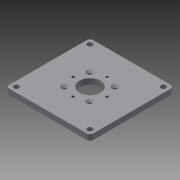
# Autodesk Inventor part: base_mount
Saved by Autodesk Inventor 2015 (Build 190159000, 159)
## iProperties
Created: 2015-12-01
Part Number: base_mount
Material: Generic
Document SubType Name: Modeling
Designer: jufranz
Density: 1 g/cm^3
Appearance: Default
Author: jufranz
Autodesk Inventor part; units mm, degrees
ref_plane "YZ Plane" through (0, 0, 0) normal (1, 0, 0) x (0, 1, 0)
ref_plane "XZ Plane" through (0, 0, 0) normal (0, 1, 0) x (-1, 0, 0)
ref_plane "XY Plane" through (0, 0, 0) normal (0, 0, 1) x (1, 0, 0)
sketch "Sketch1" plane through (0, 0, 0) normal (0, 1, 0) x (-1, 0, 0)
  line L0 (40, 36.825) -> (40, -36.825)
  line L1 (36.825, -40) -> (-36.825, -40)
  line L2 (-40, -36.825) -> (-40, 36.825)
  line L3 (-36.825, 40) -> (-13.175, 40)
  line L4 (13.175, 40) -> (36.825, 40)
  arc A0 (40, 36.825) -> (36.825, 40) centre (36.825, 36.825) ccw
  arc A1 (36.825, -40) -> (40, -36.825) centre (36.825, -36.825) ccw
  arc A2 (-40, -36.825) -> (-36.825, -40) centre (-36.825, -36.825) ccw
  arc A3 (-36.825, 40) -> (-40, 36.825) centre (-36.825, 36.825) ccw
  line L5 (13.175, 40) -> (-13.175, 40)
  point P0 (0, 0)
  point P1 (40, 40)
  point P2 (40, -40)
  point P3 (-40, -40)
  point P4 (-40, 40)
  point P5 (-10, 40)
  point P6 (10, 40)
  point P7 (40, 0)
  point P8 (0, -40)
  point P9 (0, 60)
  dimension "d0" = 80
  dimension "d1" = 80
  dimension "d27" = 3.175
  constraints: 12 end point, 11 point on line, 8 point on circle, 8 tangent, 4 centre point, 3 equal radius, 3 perpendicular, 2 midpoint, 2 vertical alignment, 1 horizontal, 1 horizontal alignment, 1 vertical
  measures "d0" distance of point (40, 40) point (40, -40)
  measures "d1" distance of point (40, -40) point (-40, -40)
  measures "d27" radius of A0
extrude "Extrusion1" add sketch "Sketch1" along normal blind 5.334
sketch "Sketch2" plane through (0, 5.334, 0) normal (0, 1, 0) x (1, 0, 0)
  line L0 (-12.0208, -12.0208) -> (0, 0)
  line L1 (0, 0) -> (-40, 0)
  line L2 (-40, 36.825) -> (-40, -36.825) projected
  point P0 (-17.5, 17.5)
  point P1 (-17.5, -17.5)
  point P2 (12.0208, -12.0208)
  point P3 (12.0208, 12.0208)
  point P4 (-12.0208, 12.0208)
  dimension "d6" = 17
  dimension "d7" = 45
  dimension "d10" = 360
  constraints: 4 end point, 1 coincident, 7 other
  measures "d6" distance of point (0, 0) L0.start
  measures "d7" angle of L0 L1
hole "Hole1" at (-12.0208, 5.334, 12.0208) at (12.0208, 5.334, 12.0208) at (12.0208, 5.334, -12.0208) at (-12.0208, 5.334, -12.0208) direction (0, -1, 0) diameter 3.2 end through all countersink diameter 6.35 countersink angle 82
sketch "Sketch3" plane through (0, 5.334, 0) normal (0, 1, 0) x (1, 0, 0)
  point P0 (0, 0)
  point P1 (0, 0)
  constraints: 1 coincident
hole "Hole2" at (0, 5.334, 0) direction (0, -1, 0) diameter 20 end through all
sketch "Sketch4" plane through (0, 5.334, 0) normal (0, 1, 0) x (1, 0, 0)
  point P0 (0, 0)
  point P1 (-16.215, 0)
  point P2 (0, -16.215)
  point P3 (16.215, 0)
  point P4 (0, 16.215)
  dimension "d29" = 16.215
  dimension "d47" = 360
  constraints: 5 other
  measures "d29" distance of point (-16.215, 0) point (0, 0)
hole "Hole3" at (-16.215, 5.334, 0) at (0, 5.334, 16.215) at (16.215, 5.334, 0) at (0, 5.334, -16.215) direction (0, -1, 0) diameter 2.4638 end through all
sketch "Sketch7" plane through (0, 5.334, 0) normal (0, 1, 0) x (1, 0, 0)
  line L0 (-40, 36.825) -> (-40, -36.825) projected
  line L1 (36.825, 40) -> (-36.825, 40) projected
  line L2 (-36.825, -40) -> (36.825, -40) projected
  line L3 (40, -36.825) -> (40, 36.825) projected
  point P0 (0, 0)
  point P1 (-35, 35)
  point P2 (35, 35)
  point P3 (35, -35)
  point P4 (-35, -35)
  dimension "d49" = 5
  dimension "d50" = 5
  dimension "d51" = 5
  dimension "d52" = 5
  constraints: 2 horizontal alignment, 2 vertical alignment
  measures "d49" distance from line of L0 point (-35, 35)
  measures "d50" distance from line of point (-35, 35) L1
  measures "d51" distance from line of L2 point (-35, -35)
  measures "d52" distance from line of L3 point (35, 35)
hole "Hole4" at (-35, 5.334, -35) at (35, 5.334, -35) at (35, 5.334, 35) at (-35, 5.334, 35) direction (0, -1, 0) diameter 5 end through all
equation "\"d50\" = d49"
equation "\"d51\" = d49"
equation "\"d52\" = d49"
body "Solid1"
